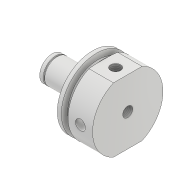
# Autodesk Inventor part: soporte planetario
Saved by Autodesk Inventor 2022 (Build 260153000, 153)
## iProperties
Created: 2019-06-06
Part Number: soporte planetario
Material: Acetal Resin, Black
Document SubType Name: Modeling
Designer: usuario_2
Density: 1.425 g/cm^3
Appearance: Blanco
Mass: 159.043 g
Surface Area: 243.105 cm^2
Volume: 140.746 cm^3
Author: usuario_2
Autodesk Inventor part; units mm, degrees
ref_plane "YZ Plane" through (0, 0, 0) normal (1, 0, 0) x (0, 1, 0)
sketch "Boceto1" plane through (0, 0, 0) normal (0, 0, 1) x (1, 0, 0)
  line L0 (40, 35) -> (44, 35)
  line L1 (75, 35) -> (75, 0)
  line L2 (40, 12.5) -> (40, 15) construction
  line L3 (0, 0) -> (75, 0)
  line L4 (40, 15) -> (30, 15)
  line L5 (30, 15) -> (30, 12.5)
  line L6 (30, 12.5) -> (40, 12.5) construction
  line L7 (40, 15) -> (40, 35)
  line L8 (3.5, 12.5) -> (3.5, 11.5)
  line L9 (3.5, 11.5) -> (5, 11.5)
  line L10 (5, 11.5) -> (5, 12.5)
  line L11 (5, 12.5) -> (30, 12.5)
  line L12 (3.5, 12.5) -> (5, 12.5) construction
  line L13 (0, 12.5) -> (0, 0)
  line L14 (0, 12.5) -> (3.5, 12.5)
  line L15 (65, 35) -> (65, 0) construction
  line L16 (44, 35) -> (45.3397, 30)
  line L17 (45.3397, 30) -> (49.3397, 30)
  line L18 (49.3397, 30) -> (50.6795, 35)
  line L19 (47.3397, 30) -> (47.3397, 35) construction
  line L20 (47.3397, 35) -> (50.6795, 35) construction
  line L21 (44, 35) -> (47.3397, 35) construction
  line L22 (50.6795, 35) -> (75, 35)
  dimension "d59" = 75
  dimension "d61" = 35
  dimension "d82" = 35
  dimension "d111" = 10
  dimension "d112" = 15
  dimension "d113" = 1.5
  dimension "d114" = 1
  dimension "d115" = 25
  dimension "d130" = 12.5
  dimension "d133" = 10
  dimension "d134" = 2
  dimension "d135" = 105
  dimension "d136" = 105
  dimension "d137" = 5
  dimension "d138" = 4
  constraints: 46 end point, 18 perpendicular, 7 horizontal, 7 point on line, 5 vertical, 1 midpoint
  measures "d59" distance from line of L13.end L1
  measures "d61" distance from line of L2.start L1
  measures "d82" distance of L1.start L1.end
  measures "d111" distance of L2.end L4.end
  measures "d112" distance between parallel lines of L3 L4
  measures "d113" distance of L8.end L9.end
  measures "d114" distance of L8.start L8.end
  measures "d115" distance between parallel lines of L5 L10
  measures "d130" distance between parallel lines of L3 L14
  measures "d133" distance between parallel lines of L1 L15
  measures "d134" distance from line of L16.end L19
  measures "d135" angle of L17 L16
  measures "d136" angle of L17 L18
  measures "d137" distance between parallel lines of L0 L17
  measures "d138" distance of L0.start L0.end
revolve "Revolución1" add sketch "Boceto1" angle 360 about axis through (0, 0, 0) along (1, 0, 0)
ref_plane "Plano de trabajo3" through (0, 0, 15) normal (0, 0, 1) x (1, 0, 0)
sketch "Boceto3" plane through (0, 0, 15) normal (0, 0, 1) x (1, 0, 0)
  circle A0 centre (63, 0) radius 5
  line L0 (75, -35) -> (75, 35) projected
  point P0 (0, 0)
  dimension "d14" = 5
  dimension "d132" = 12
  constraints: 1 centre point, 1 horizontal alignment
  measures "d14" radius of A0
  measures "d132" distance from line of L0 A0.centre
extrude "Extrusión1" cut sketch "Boceto3" along normal blind 80
mirror "Simetría1" about plane through (0, 0, 0) normal (0, 0, 1) of "Extrusión1"
sketch "Boceto10" plane through (75, 0, 0) normal (1, 0, 0) x (0, 0, -1)
  circle A0 centre (0, 0) radius 45.5
  circle A1 centre (0, 0) radius 12.5 construction
  circle A2 centre (0, 0) radius 5
  dimension "d116" = 91
  dimension "d117" = 10
  constraints: 2 centre point, 1 coincident, 1 concentric
  measures "d116" diameter of A0
  measures "d117" diameter of A2
extrude "Extrusión11" cut sketch "Boceto10" against normal blind 20 contours A2
thread "Rosca5"
thread "Rosca6"
thread "Rosca7"
ref_plane "Plano de trabajo6" through (62.8397, -35, 0) normal (0, 1, 0) x (-1, 0, 0)
sketch "Boceto15" plane through (62.8397, -35, 0) normal (0, 1, 0) x (-1, 0, 0)
  circle A0 centre (-0.1603, 0) radius 5
  line L0 (-12.1603, 35) -> (-12.1603, -35) projected
  point P0 (62.8397, 0)
  dimension "d139" = 10
  dimension "d140" = 12
  constraints: 1 centre point, 1 horizontal alignment
  measures "d139" diameter of A0
  measures "d140" distance from line of L0 A0.centre
sketch "Boceto16" plane through (0, 0, 0) normal (0, 0, 1) x (1, 0, 0)
  line L0 (50.6795, -35) -> (75, -35) projected
  line L1 (62.8397, -35) -> (29.2758, 5)
  line L2 (62.8397, -35) -> (62.8397, 5) construction
  point P0 (0, 0)
  dimension "d141" = 40
  dimension "d151" = 5
  constraints: 4 end point, 1 midpoint, 1 perpendicular
  measures "d141" angle of L2 L1
  measures "d151" vertical distance of point (0, 0) L1.end
sweep "Barrido1" cut profiles "Boceto15" path "Boceto16" path curves L1
sketch "Boceto17" plane through (0, 0, 0) normal (-1, 0, 0) x (0, 0, 1)
  circle A0 centre (0, 0) radius 5 projected
  circle A1 centre (0, 0) radius 5
  point P0 (0, 0)
  dimension "d144" = 10
  constraints: 1 centre point, 1 coincident
  measures "d144" diameter of A1
extrude "Extrusión13" cut sketch "Boceto17" against normal up to surface
sketch "Sketch18" plane through (75, 0, 0) normal (1, 0, 0) x (0, 0, -1)
  circle A0 centre (0, 0) radius 35 projected
  line L0 (-32, -14.1774) -> (-32, 14.1774)
  line L1 (32, -14.1774) -> (32, 14.1774)
  point P0 (0, 0)
  dimension "d152" = 32
  dimension "d153" = 32
  constraints: 4 end point, 4 point on circle, 2 vertical
  measures "d152" distance from line of A0.centre L0
  measures "d153" distance from line of point (0, 0) L1
extrude "Extrusion14" cut sketch "Sketch18" against normal blind 25 contours A0 L1 | L0 A0
